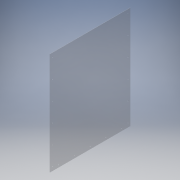
# Autodesk Inventor part: Short Wall
Saved by Autodesk Inventor 2017 (Build 210142000, 142)
## iProperties
Created: 2017-01-16
Part Number: Short Wall
Material: Polycarbonate, Clear
Document SubType Name: Modeling
Designer: Ben
Density: 1.2 g/cm^3
Appearance: Polycarbonate - Clear
Mass: 263.627 g
Surface Area: 2791.53 cm^2
Volume: 219.689 cm^3
Author: Ben
Autodesk Inventor part; units mm, degrees
ref_plane "YZ Plane" through (0, 0, 0) normal (1, 0, 0) x (0, 1, 0)
ref_plane "XZ Plane" through (0, 0, 0) normal (0, 1, 0) x (-1, 0, 0)
ref_plane "XY Plane" through (0, 0, 0) normal (0, 0, 1) x (1, 0, 0)
sketch "Sketch1" plane through (0, 0, 0) normal (1, 0, 0) x (0, 1, 0)
  line L0 (0, 0) -> (412.75, 0)
  line L1 (412.75, 0) -> (412.75, -323.85)
  line L2 (412.75, -323.85) -> (0, -323.85)
  line L3 (0, -323.85) -> (0, 0)
  line L4 (0, -314.325) -> (412.75, -314.325) construction
  line L5 (412.75, -161.925) -> (0, -161.925) construction
  line L6 (206.375, -323.85) -> (206.375, 0) construction
  circle A0 centre (15.875, -314.325) radius 1.5875
  circle A1 centre (92.075, -314.325) radius 1.5875
  circle A2 centre (168.275, -314.325) radius 1.5875
  circle A3 centre (244.475, -314.325) radius 1.5875
  circle A4 centre (320.675, -314.325) radius 1.5875
  circle A5 centre (396.875, -314.325) radius 1.5875
  line L7 (0, -9.525) -> (412.75, -9.525) construction
  circle A6 centre (15.875, -9.525) radius 1.5875
  circle A7 centre (92.075, -9.525) radius 1.5875
  circle A8 centre (168.275, -9.525) radius 1.5875
  circle A9 centre (244.475, -9.525) radius 1.5875
  circle A10 centre (320.675, -9.525) radius 1.5875
  circle A11 centre (396.875, -9.525) radius 1.5875
  line L8 (9.525, -323.85) -> (9.525, 0) construction
  circle A12 centre (9.525, -161.925) radius 1.5875
  circle A13 centre (9.525, -98.425) radius 1.5875
  circle A14 centre (9.525, -34.925) radius 1.5875
  circle A15 centre (9.525, -225.425) radius 1.5875
  circle A16 centre (9.525, -161.925) radius 1.5875
  circle A17 centre (9.525, -98.425) radius 1.5875
  circle A18 centre (9.525, -288.925) radius 1.5875
  circle A19 centre (9.525, -225.425) radius 1.5875
  circle A20 centre (9.525, -161.925) radius 1.5875
  dimension "d0" = 323.85
  dimension "d1" = 412.75
  dimension "d4" = 3.175
  dimension "d7" = 76.2
  dimension "d12" = 9.525
  dimension "d13" = 9.525
  dimension "d16" = 63.5
  dimension "d19" = 63.5
  constraints: 21 centre point, 18 end point, 8 symmetric about line, 6 point on line, 5 midpoint, 3 perpendicular, 2 horizontal, 2 parallel, 2 vertical, 1 equal radius, 33 other
  measures "d0" distance of L2.end L0.start
  measures "d1" distance of L0.start L0.end
  measures "d4" diameter of A0
  measures "d7" distance of A0.centre A1.centre
  measures "d12" distance between parallel lines of L2 L4
  measures "d13" distance between parallel lines of L3 L8
  measures "d16" distance of A12.centre A13.centre
  measures "d19" distance of A12.centre A15.centre
extrude "Extrusion1" add sketch "Sketch1" along normal blind 1.5875
equation "\"d13\" = d12"
body "Solid1"
